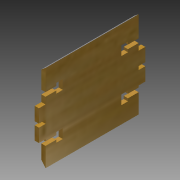
# Autodesk Inventor part: lat_front_mdf
Saved by Autodesk Inventor 2014 (Build 180170000, 170)
## iProperties
Created: 2015-01-29
Part Number: lat_front_mdf
Material: Generic
Document SubType Name: Modeling
Designer: Gabriel
Density: 1 g/cm^3
Appearance: Default
Author: Gabriel
Autodesk Inventor part; units mm, degrees
ref_plane "YZ Plane" through (0, 0, 0) normal (1, 0, 0) x (0, 1, 0)
ref_plane "XZ Plane" through (0, 0, 0) normal (0, 1, 0) x (-1, 0, 0)
ref_plane "XY Plane" through (0, 0, 0) normal (0, 0, 1) x (1, 0, 0)
sketch "Sketch3" plane through (0, 0, 0) normal (0, 1, 0) x (-1, 0, 0)
  line L0 (0, 0) -> (0, -64.031)
  line L1 (0, -64.031) -> (3.1235, -60.1267)
  line L2 (0, -64.031) -> (3.1235, -60.1267)
  line L3 (3.1235, -60.1267) -> (3.1235, -2.4988)
  line L4 (0, 0) -> (3.1235, -2.4988)
  line L5 (3.1235, -2.4988) -> (0, -2.4988)
  line L6 (0, -2.4988) -> (0, -12.4988)
  line L7 (3.1235, -2.4988) -> (3.1235, -12.4988)
  line L8 (3.1235, -60.1267) -> (0, -60.1267)
  line L9 (3.1235, -60.1267) -> (3.1235, -50.1267)
  line L10 (0, 0) -> (0, -20)
  line L11 (0, -64.031) -> (0, -48.031)
  line L12 (0, -50.1267) -> (0, -48.031)
  line L13 (0, -20) -> (0, -30)
  line L14 (0, -60.1267) -> (0, -45.1267)
  line L15 (0, -45.1267) -> (3.1235, -45.1267)
  line L16 (0, -45.1267) -> (0, -35.1267)
  line L17 (0, -35.1267) -> (3.1235, -35.1267)
  line L18 (0, -2.4988) -> (0, -22.4988)
  line L19 (0, -22.4988) -> (3.1235, -22.4988)
  line L20 (0, -22.4988) -> (0, -32.4988)
  line L21 (0, -32.4988) -> (3.1235, -32.4988)
  line L22 (0, 0) -> (0, -16)
  line L23 (0, -16) -> (3.1235, -16)
  line L24 (0, -64.031) -> (0, -48.031)
  line L25 (0, -48.031) -> (3.1235, -48.031)
  line L26 (0, -48.031) -> (0, -45.1267)
  line L27 (3.1235, -22.4988) -> (3.1235, -16)
  line L28 (3.1235, -2.4988) -> (3.1235, -1.1988)
  line L29 (3.1235, -1.1988) -> (0, 1.3)
  line L30 (0, 1.3) -> (0, 0)
  point P0 (3.1235, -20)
  point P1 (3.1235, -30)
  dimension "d80" = 15
  dimension "d81" = 10
  dimension "d86" = 20
  dimension "d87" = 10
  dimension "d90" = 16
  dimension "d91" = 16
  dimension "d92" = 2.9043
  dimension "d93" = 6.4988
  dimension "d96" = 1.3
  constraints: 58 end point, 7 horizontal, 3 collinear, 3 vertical, 2 parallel, 2 perpendicular, 2 point on line, 26 other
  measures "d80" distance of L8.end L14.end
  measures "d81" distance of L14.end L16.end
  measures "d86" distance of L5.end L18.end
  measures "d87" distance of L18.end L20.end
  measures "d90" distance of L4.start L22.end
  measures "d91" distance of L1.start L11.end
  measures "d92" distance of L11.end L14.end
  measures "d93" distance of L19.end L23.end
  measures "d96" distance of L4.end L28.end
extrude "Extrusion4" add sketch "Sketch3" along normal blind 70 contours L4 L5 L0 | L5 L3 L23 L0 | L23 L3 L19 L0 | L3 L21 L0 L19 | L3 L17 L0 L21 | L3 L15 L0 L17 | L3 L25 L0 L15 | L3 L8 L0 L25 | L1 L0 L8
sketch "Sketch4" plane through (0, 0, 0) normal (1, 0, 0) x (0, 0, -1)
  line L0 (0, 0) -> (16, 0)
  line L1 (16, 0) -> (48, 0)
  line L2 (48, 0) -> (64, 0)
  line L3 (16, 0) -> (14.5, 0)
  line L4 (14.5, 0) -> (14.5, 8)
  line L5 (14.5, 8) -> (12.5, 8)
  line L6 (12.5, 8) -> (12.5, 13)
  line L7 (12.5, 13) -> (19.5, 13)
  line L8 (19.5, 13) -> (19.5, 8)
  line L9 (19.5, 8) -> (17.5, 8)
  line L10 (16, 0) -> (17.5, 0)
  line L11 (17.5, 0) -> (17.5, 8)
  line L12 (48, 0) -> (49.5, 0)
  line L13 (48, 0) -> (46.5, 0)
  line L14 (48, 0) -> (46.5, 0)
  line L15 (46.5, 0) -> (46.5, 8)
  line L16 (46.5, 8) -> (44.5, 8)
  line L17 (44.5, 8) -> (44.5, 13)
  line L18 (44.5, 13) -> (51.5, 13)
  line L19 (51.5, 13) -> (51.5, 8)
  line L20 (51.5, 8) -> (49.5, 8)
  line L21 (49.5, 8) -> (49.5, 0)
  line L22 (16, 13) -> (16, 57)
  line L23 (16, 70) -> (17.5, 70)
  line L24 (17.5, 70) -> (17.5, 62)
  line L25 (17.5, 62) -> (19.5, 62)
  line L26 (19.5, 62) -> (19.5, 57)
  line L27 (19.5, 57) -> (12.5, 57)
  line L28 (12.5, 57) -> (12.5, 62)
  line L29 (12.5, 62) -> (14.5, 62)
  line L30 (14.5, 62) -> (14.5, 70)
  line L31 (48, 13) -> (48, 57)
  line L32 (48, 70) -> (49.5, 70)
  line L33 (49.5, 70) -> (49.5, 62)
  line L34 (49.5, 62) -> (51.5, 62)
  line L35 (51.5, 62) -> (51.5, 57)
  line L36 (51.5, 57) -> (44.5, 57)
  line L37 (44.5, 57) -> (44.5, 62)
  line L38 (44.5, 62) -> (46.5, 62)
  line L39 (46.5, 62) -> (46.5, 70)
  line L40 (46.5, 70) -> (48, 70)
  line L41 (16, 70) -> (14.5, 70)
  dimension "d23" = 16
  dimension "d24" = 32
  dimension "d25" = 16
  dimension "d26" = 1.5
  dimension "d27" = 8
  dimension "d28" = 2
  dimension "d29" = 5
  dimension "d30" = 7
  dimension "d31" = 2
  dimension "d32" = 1.5
  dimension "d33" = 1.5
  dimension "d34" = 1.5
  dimension "d35" = 1.5
  dimension "d36" = 8
  dimension "d37" = 2
  dimension "d38" = 7
  dimension "d39" = 70
  dimension "d40" = 8
  dimension "d41" = 2
  dimension "d42" = 5
  dimension "d43" = 7
  dimension "d44" = 5
  dimension "d45" = 1.5
  dimension "d46" = 8
  dimension "d47" = 2
  constraints: 84 end point, 21 parallel, 9 perpendicular, 6 collinear, 4 midpoint, 4 point on line, 1 horizontal
  measures "d23" distance of L0.start L0.end
  measures "d24" distance of L0.end L1.end
  measures "d25" distance of L1.end L2.end
  measures "d26" distance of L0.end L3.end
  measures "d27" distance of L3.end L4.end
  measures "d28" distance of L4.end L5.end
  measures "d29" distance of L5.end L6.end
  measures "d30" distance of L6.end L7.end
  measures "d31" distance of L8.end L9.end
  measures "d32" distance of L0.end L10.end
  measures "d33" distance of L1.end L12.end
  measures "d34" distance of L1.end L13.end
  measures "d35" distance of L1.end L13.end
  measures "d36" distance of L13.end L15.end
  measures "d37" distance of L15.end L16.end
  measures "d38" distance of L17.end L18.end
  measures "d39" distance of L0.end L23.start
  measures "d40" distance of L23.end L24.end
  measures "d41" distance of L24.end L25.end
  measures "d42" distance of L25.end L26.end
  measures "d43" distance of L26.end L27.end
  measures "d44" distance of L27.end L28.end
  measures "d45" distance of L32.start L32.end
  measures "d46" distance of L32.end L33.end
  measures "d47" distance of L33.end L34.end
extrude "Extrusion5" cut sketch "Sketch4" against normal blind 3.2 contours L4 L5 L6 L7 L8 L9 L11 L1 L0
extrude "Extrusion6" cut sketch "Sketch4" against normal blind 3.2 contours L15 L16 L17 L18 L19 L20 L21 L2 L1
extrude "Extrusion7" cut sketch "Sketch4" against normal blind 3.2 contours L36 L37 L38 L39 L40 L32 L33 L34 L35
extrude "Extrusion8" cut sketch "Sketch4" against normal blind 3.2 contours L27 L28 L29 L30 L41 L23 L24 L25 L26
sketch "Sketch6" plane through (0, 70, 0) normal (0, 1, 0) x (1, 0, 0)
  line L0 (0, 0) -> (0, 2.499)
  line L1 (-3.123, 2.499) -> (-3.123, 12.499)
  line L2 (0, 12.499) -> (0, 2.499)
  line L3 (0, 0) -> (0, 64)
  line L4 (0, 2.499) -> (0, 60.127)
  line L5 (-3.123, 55.127) -> (-3.123, 45.127)
  line L6 (-3.123, 55.127) -> (-3.123, 40.127)
  line L7 (-3.123, 40.127) -> (-3.123, 30.127)
  line L8 (0, 30.127) -> (0, 40.127)
  line L9 (-3.123, 60.127) -> (0, 60.127)
  line L10 (-3.123, 60.127) -> (-3.123, 45.127)
  line L11 (-3.123, 45.127) -> (0, 45.127)
  line L12 (-3.123, 45.127) -> (-3.123, 35.127)
  line L13 (-3.123, 35.127) -> (0, 35.127)
  line L14 (0, 35.127) -> (0, 45.127)
  line L15 (-3.123, 2.499) -> (0, 2.499)
  line L16 (-3.123, 2.499) -> (-3.123, 22.499)
  line L17 (-3.123, 22.499) -> (0, 22.499)
  line L18 (-3.123, 22.499) -> (-3.123, 32.499)
  line L19 (-3.123, 32.499) -> (0, 32.499)
  line L20 (0, 32.499) -> (0, 22.499)
  line L21 (-3.123, 2.3854) -> (-3.123, 1.3854)
  line L22 (-2.9831, 1.2495) -> (0, -1.1378)
  line L23 (-2.9831, 1.2495) -> (0.8377, 1.2495) construction
  line L24 (0, -1.1378) -> (0, 0)
  dimension "d63" = 3.123
  dimension "d65" = 64
  dimension "d75" = 15
  dimension "d76" = 10
  dimension "d77" = 20
  dimension "d78" = 10
  dimension "d94" = 1
  dimension "d95" = 38.67
  constraints: 50 end point, 8 point on line, 7 perpendicular, 5 collinear, 3 parallel, 2 midpoint, 1 equal length, 1 horizontal, 1 vertical
  measures "d63" distance of L0.end L1.start
  measures "d65" distance of L0.start L3.end
  measures "d75" distance of L9.start L5.end
  measures "d76" distance of L5.end L12.end
  measures "d77" distance of L1.start L16.end
  measures "d78" distance of L16.end L18.end
  measures "d94" distance of L21.start L21.end
  measures "d95" angle of L22 L23
extrude "Extrusion13" add sketch "Sketch6" along normal blind 5 contours L18 L7 L19 L3 L17 | L7 L6 L11 L3 L13
extrude "Extrusion14" add sketch "Sketch3" against normal blind 5 contours L3 L21 L0 L19 | L3 L15 L0 L17
extrude "Extrusion15" add sketch "Sketch3" along normal blind 70 contours L30 L29 L28 L4
body "Solid4"
